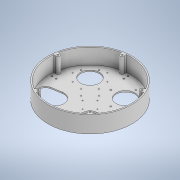
# Autodesk Inventor part: RL_spider_center_mid_v3
Saved by Autodesk Inventor 2022 (Build 260153000, 153)
## iProperties
Created: 2021-08-09
Part Number: RL_spider_center_mid_v3
Material: Generic
Document SubType Name: Modeling
Designer: james
Density: 1 g/cm^3
Appearance: Default
Author: james
Autodesk Inventor part; units mm, degrees
ref_plane "YZ Plane" through (0, 0, 0) normal (1, 0, 0) x (0, 1, 0)
ref_plane "XZ Plane" through (0, 0, 0) normal (0, 1, 0) x (-1, 0, 0)
ref_plane "XY Plane" through (0, 0, 0) normal (0, 0, 1) x (1, 0, 0)
sketch "Sketch1" plane through (0, 0, 0) normal (0, 1, 0) x (-1, 0, 0)
  circle A0 centre (0, 0) radius 100
  dimension "d0" = 200
  constraints: 1 centre point, 1 coincident
  measures "d0" diameter of A0
extrude "Extrusion1" add sketch "Sketch1" along normal blind 40
sketch "Sketch3" plane through (0, 40, 0) normal (0, 1, 0) x (1, 0, 0)
  circle A0 centre (0, 0) radius 97
  circle A1 centre (0, 0) radius 100 projected
  dimension "d14" = 3
  constraints: 1 centre point, 1 coincident
  measures "d14" radial gap between concentric circles of A0 A1
extrude "Extrusion3" cut sketch "Sketch3" against normal blind 37 contours A0
sketch "Sketch6" plane through (0, 40, 0) normal (0, 1, 0) x (1, 0, 0)
  circle A0 centre (65.0538, -65.0538) radius 2.2
  line L0 (0, 0) -> (65.0538, -65.0538)
  line L1 (0, 0) -> (0, 29.3697)
  arc A1 (68.5894, -61.5183) -> (61.5183, -68.5894) centre (65.0538, -65.0538) ccw
  line L2 (61.5183, -68.5894) -> (64.9626, -72.0337)
  line L3 (68.5894, -61.5183) -> (72.0337, -64.9626)
  arc A2 (79.7026, 46.2222) -> (84.2426, 37.3121) centre (81.9726, 41.7671) ccw
  circle A3 centre (81.9726, 41.7671) radius 2.2
  line L4 (84.2426, 37.3121) -> (88.5827, 39.5235)
  line L5 (79.7026, 46.2222) -> (84.0428, 48.4336)
  arc A4 (-19.3304, 90.0852) -> (-9.4535, 91.6495) centre (-14.392, 90.8673) ccw
  circle A5 centre (-14.392, 90.8673) radius 2.2
  line L6 (-9.4535, 91.6495) -> (-10.2155, 96.4606)
  line L7 (-19.3304, 90.0852) -> (-20.0924, 94.8962)
  arc A6 (-91.6495, 9.4535) -> (-90.0852, 19.3304) centre (-90.8673, 14.392) ccw
  circle A7 centre (-90.8673, 14.392) radius 2.2
  line L8 (-90.0852, 19.3304) -> (-94.8962, 20.0924)
  line L9 (-91.6495, 9.4535) -> (-96.4606, 10.2155)
  arc A8 (-37.3121, -84.2426) -> (-46.2222, -79.7026) centre (-41.7671, -81.9726) ccw
  circle A9 centre (-41.7671, -81.9726) radius 2.2
  line L10 (-46.2222, -79.7026) -> (-48.4336, -84.0428)
  line L11 (-37.3121, -84.2426) -> (-39.5235, -88.5827)
  circle A10 centre (0, 0) radius 97 projected
  dimension "d106" = 4.4
  dimension "d109" = 92
  dimension "d111" = 135
  dimension "d112" = 10
  dimension "d115" = 360
  constraints: 24 end point, 10 centre point, 10 point on circle, 2 coincident, 2 parallel, 2 tangent, 1 vertical, 52 other
  measures "d106" diameter of A0
  measures "d109" distance of A0.centre L0.start
  measures "d111" angle of L0 L1
  measures "d112" diameter of A1
extrude "Extrusion6" add sketch "Sketch6" against normal up to surface (37 mm away) contours A1 L3 A10 L2 | A10 L10 A8 L11 | L4 A2 L5 A10 | A10 L8 A6 L9 | L6 A4 L7 A10
sketch "Sketch9" plane through (0, 3, 0) normal (0, 1, 0) x (1, 0, 0)
  circle A0 centre (37.4767, 71.4178) radius 1.75
  circle A1 centre (7.7782, 41.7193) radius 1.75
  circle A2 centre (71.4178, 37.4767) radius 1.75
  circle A3 centre (41.7193, 7.7782) radius 1.75
  line L0 (0, 0) -> (0, 0)
  line L1 (0, 0) -> (-23.1827, 0)
  line L2 (0, 0) -> (0, 0)
  dimension "d115" = 360
  dimension "d77" = 42
  dimension "d78" = 48
  dimension "d79" = 42
  dimension "d80" = 48
  dimension "d81" = 135
  dimension "d82" = 24
  dimension "d83" = 24
  dimension "d84" = 24
  dimension "d85" = 3.5
  dimension "d86" = 3.5
  dimension "d87" = 3.5
  dimension "d88" = 3.5
  dimension "d89" = 35
  constraints: 6 end point, 4 centre point, 1 horizontal, 1 perpendicular
  measures "d77" distance of A1.centre A0.centre
  measures "d78" distance of A3.centre A1.centre
  measures "d79" distance of A3.centre A2.centre
  measures "d80" distance of A2.centre A0.centre
  measures "d81" angle of L0 L1
  measures "d82" distance from line of L0 A1.centre
  measures "d83" distance from line of A3.centre L0
  measures "d84" distance from line of L0 A0.centre
  measures "d85" diameter of A1
  measures "d86" diameter of A3
  measures "d87" diameter of A0
  measures "d88" diameter of A2
  measures "d89" distance from line of L2 A1.centre
extrude "Extrusion9" cut sketch "Sketch9" against normal blind 4
sketch "Sketch18" plane through (0, 3, 0) normal (0, 1, 0) x (1, 0, 0)
  line L0 (54.624, -13.2583) -> (13.2583, -54.624)
  line L1 (13.2583, -54.624) -> (31.643, -73.0088)
  line L2 (31.643, -73.0088) -> (73.0088, -31.643)
  line L3 (73.0088, -31.643) -> (54.624, -13.2583)
  line L4 (0, 0) -> (3.812, 0)
  line L5 (0, 0) -> (33.9411, -33.9411)
  circle A0 centre (54.624, -13.2583) radius 1.15
  circle A1 centre (73.0088, -31.643) radius 1.15
  circle A2 centre (13.2583, -54.624) radius 1.15
  circle A3 centre (31.643, -73.0088) radius 1.15
  line L6 (3.5355, -49.4975) -> (36.7696, -82.7315)
  line L7 (36.7696, -82.7315) -> (82.7315, -36.7696)
  line L8 (82.7315, -36.7696) -> (49.4975, -3.5355)
  line L9 (49.4975, -3.5355) -> (3.5355, -49.4975)
  dimension "d193" = 45
  dimension "d194" = 2.3
  dimension "d195" = 2.3
  dimension "d196" = 2.3
  dimension "d197" = 2.3
  dimension "d198" = 48
  dimension "d199" = 26
  dimension "d200" = 58.5
  dimension "d201" = 47
  dimension "d202" = 10.5
  dimension "d203" = 65
  dimension "d204" = 32.5
  constraints: 20 end point, 7 perpendicular, 4 centre point, 4 coincident, 1 horizontal, 1 midpoint
  measures "d193" angle of L4 L5
  measures "d194" diameter of A0
  measures "d195" diameter of A1
  measures "d196" diameter of A2
  measures "d197" diameter of A3
  measures "d198" distance of L4.start L5.end
  measures "d199" distance of L2.end L0.start
  measures "d200" distance of L1.end L2.end
  measures "d201" distance of L6.start L6.end
  measures "d202" distance between parallel lines of L0 L9
  measures "d203" distance of L8.end L6.start
  measures "d204" distance between parallel lines of L5 L6
extrude "Extrusion11" cut sketch "Sketch18" against normal blind 10 contours L3 A0 L0 | L0 A0 L3 | A1 L2 L3 | L3 L2 A1 | A2 L1 L0 | L0 L1 A2 | A3 L1 L2 | L2 L1 A3
sketch "Sketch12" plane through (0, 3, 0) normal (0, 1, 0) x (1, 0, 0)
  circle A0 centre (-73.0088, 31.643) radius 1.15
  circle A1 centre (-54.624, 13.2583) radius 1.15
  circle A2 centre (-31.643, 73.0088) radius 1.15
  circle A3 centre (-13.2583, 54.624) radius 1.15
  line L0 (-54.624, 13.2583) -> (-73.0088, 31.643)
  line L1 (-73.0088, 31.643) -> (-31.643, 73.0088)
  line L2 (-31.643, 73.0088) -> (-13.2583, 54.624)
  line L3 (-13.2583, 54.624) -> (-54.624, 13.2583)
  line L4 (0, 0) -> (-33.9411, 33.9411)
  line L5 (0, 0) -> (28.9474, 0)
  line L6 (-3.5355, 49.4975) -> (-49.4975, 3.5355)
  line L7 (-49.4975, 3.5355) -> (-82.7315, 36.7696)
  line L8 (-82.7315, 36.7696) -> (-36.7696, 82.7315)
  line L9 (-36.7696, 82.7315) -> (-3.5355, 49.4975)
  dimension "d132" = 135
  dimension "d133" = 58.5
  dimension "d134" = 26
  dimension "d135" = 48
  dimension "d138" = 2.3
  dimension "d139" = 2.3
  dimension "d140" = 2.3
  dimension "d141" = 2.3
  dimension "d219" = 47
  dimension "d220" = 65
  dimension "d221" = 32.5
  dimension "d222" = 10.5
  constraints: 20 end point, 7 perpendicular, 4 centre point, 1 horizontal, 1 midpoint, 1 parallel
  measures "d132" angle of L4 L5
  measures "d133" distance of L2.end L0.start
  measures "d134" distance of L0.start L0.end
  measures "d135" distance of L4.start L4.end
  measures "d138" diameter of A1
  measures "d139" diameter of A0
  measures "d140" diameter of A3
  measures "d141" diameter of A2
  measures "d219" distance of L6.end L7.end
  measures "d220" distance of L6.start L6.end
  measures "d221" distance between parallel lines of L4 L7
  measures "d222" distance between parallel lines of L6 L3
extrude "Extrusion12" cut sketch "Sketch12" against normal blind 10 contours A0 L0 L1 | L1 L0 A0 | L1 L2 A2 | A2 L2 L1 | L0 L3 A1 | A1 L3 L0 | L2 L3 A3 | A3 L3 L2
sketch "Sketch13" plane through (0, 3, 0) normal (0, 1, 0) x (1, 0, 0)
  circle A0 centre (-3.8891, -13.7886) radius 1.15
  circle A1 centre (13.7886, 3.8891) radius 1.15
  circle A2 centre (13.7886, -31.4663) radius 1.15
  circle A3 centre (31.4663, -13.7886) radius 1.15
  line L0 (13.7886, 3.8891) -> (31.4663, -13.7886)
  line L1 (13.7886, 3.8891) -> (-3.8891, -13.7886)
  line L2 (-3.8891, -13.7886) -> (13.7886, -31.4663)
  line L3 (13.7886, -31.4663) -> (31.4663, -13.7886)
  line L4 (0, 0) -> (4.9497, -4.9497)
  line L5 (0, 0) -> (0, 15.8788)
  circle A4 centre (-54.624, 13.2583) radius 1.15 projected
  circle A5 centre (-13.2583, 54.624) radius 1.15 projected
  line L6 (-54.624, 13.2583) -> (-13.2583, 54.624)
  dimension "d142" = 25
  dimension "d143" = 25
  dimension "d146" = 7
  dimension "d147" = 2.3
  dimension "d148" = 2.3
  dimension "d149" = 2.3
  dimension "d150" = 2.3
  dimension "d218" = 225
  constraints: 14 end point, 4 centre point, 4 perpendicular, 1 midpoint, 1 vertical
  measures "d142" distance of L0.start L1.end
  measures "d143" distance of L0.start L0.end
  measures "d146" distance of L4.start L4.end
  measures "d147" diameter of A1
  measures "d148" diameter of A3
  measures "d149" diameter of A2
  measures "d150" diameter of A0
extrude "Extrusion13" cut sketch "Sketch13" against normal blind 10 contours A0 L2 L1 | L1 L2 A0 | L2 L3 A2 | A2 L3 L2 | L1 L0 A1 | A1 L0 L1 | L3 L0 A3 | A3 L0 L3
sketch "Sketch14" plane through (0, 3, 0) normal (0, 1, 0) x (1, 0, 0)
  circle A0 centre (-15.5563, -5.6569) radius 1.15
  circle A1 centre (-29.6985, 8.4853) radius 1.15
  circle A2 centre (5.6569, 15.5563) radius 1.15
  circle A3 centre (-8.4853, 29.6985) radius 1.15
  line L0 (-15.5563, -5.6569) -> (-29.6985, 8.4853)
  line L1 (-29.6985, 8.4853) -> (-8.4853, 29.6985)
  line L2 (-8.4853, 29.6985) -> (5.6569, 15.5563)
  line L3 (5.6569, 15.5563) -> (-15.5563, -5.6569)
  line L4 (0, 0) -> (-4.9497, 4.9497)
  line L5 (0, 0) -> (0, -29.7701)
  circle A4 centre (13.2583, -54.624) radius 1.15 projected
  circle A5 centre (54.624, -13.2583) radius 1.15 projected
  line L6 (13.2583, -54.624) -> (54.624, -13.2583)
  dimension "d153" = 20
  dimension "d154" = 30
  dimension "d155" = 2.3
  dimension "d156" = 2.3
  dimension "d157" = 2.3
  dimension "d158" = 2.3
  dimension "d160" = 7
  dimension "d217" = 225
  constraints: 14 end point, 4 centre point, 4 perpendicular, 1 midpoint, 1 vertical
  measures "d153" distance of L0.start L0.end
  measures "d154" distance of L2.end L0.start
  measures "d155" diameter of A2
  measures "d156" diameter of A3
  measures "d157" diameter of A0
  measures "d158" diameter of A1
  measures "d160" distance of L4.start L4.end
extrude "Extrusion14" cut sketch "Sketch14" against normal blind 10 contours A0 L0 L3 | L3 L0 A0 | L0 L1 A1 | A1 L1 L0 | L3 L2 A2 | A2 L2 L3 | L1 L2 A3 | A3 L2 L1
sketch "Sketch16" plane through (0, 3, 0) normal (0, 1, 0) x (1, 0, 0)
  circle A0 centre (0, 80.5) radius 1.75
  circle A1 centre (0, 90.5) radius 1.75
  circle A2 centre (0, 0) radius 100 projected
  line L0 (0, 100) -> (0, 80.5)
  dimension "d179" = 3.5
  dimension "d180" = 19.5
  dimension "d181" = 9.5
  dimension "d182" = 3.5
  constraints: 2 centre point, 2 end point, 1 vertical, 1 vertical alignment, 1 other
  measures "d179" diameter of A0
  measures "d180" distance of L0.start L0.end
  measures "d181" distance of A1.centre L0.start
  measures "d182" diameter of A1
extrude "Extrusion16" cut sketch "Sketch16" against normal blind 10 contours A0 | A1 L0 | L0 A1
pattern_circular "Circular Pattern4" count 4 over 360 about axis through (0, -10, 0) along (0, 1, 0) of "Extrusion16"
sketch "Sketch17" plane through (0, 3, 0) normal (0, 1, 0) x (1, 0, 0)
  line L0 (0, 0) -> (-53.033, -53.033)
  line L1 (-53.033, -53.033) -> (-67.1751, -38.8909)
  line L2 (0, 0) -> (-22.9121, 0)
  line L3 (0, 0) -> (-42.4264, 42.4264)
  circle A0 centre (-42.4264, 42.4264) radius 22.5
  circle A1 centre (-42.4264, -42.4264) radius 22.5
  circle A2 centre (42.4264, -42.4264) radius 22.5
  circle A3 centre (42.4264, 42.4264) radius 22.5
  line L4 (-69.6063, -24.0892) -> (-46.0732, -20.2239)
  line L5 (-73.6535, -52.4198) -> (-52.144, -62.7197)
  arc A4 (-69.6063, -24.0892) -> (-73.6535, -52.4198) centre (-67.1751, -38.8909) ccw
  point P0 (-64.8915, -41.1745)
  point P1 (-26.5165, -26.5165)
  dimension "d188" = 45
  dimension "d189" = 75
  dimension "d190" = 20
  dimension "d207" = 60
  dimension "d208" = 45
  dimension "d209" = 45
  dimension "d212" = 360
  dimension "d216" = 15
  constraints: 12 end point, 5 centre point, 4 point on circle, 4 tangent, 2 coincident, 1 horizontal, 1 perpendicular, 9 other
  measures "d188" angle of L0 L2
  measures "d189" distance of L0.start L0.end
  measures "d190" distance of L0.end L1.end
  measures "d207" distance of L0.start L3.end
  measures "d208" diameter of A0
  measures "d209" angle of L2 L3
  measures "d216" radius of A4
extrude "Extrusion18" cut sketch "Sketch17" against normal blind 10
sketch "Sketch20" plane through (0, 3, 0) normal (0, 1, 0) x (1, 0, 0)
  line L0 (0, 0) -> (-22.6274, 22.6274)
  line L1 (-22.6274, 22.6274) -> (-29.7758, 15.479)
  line L2 (-22.6274, 22.6274) -> (-15.6337, 29.6211)
  line L3 (0, 0) -> (9.6667, 0)
  circle A0 centre (-29.7758, 15.479) radius 1.75
  circle A1 centre (-15.6337, 29.6211) radius 1.75
  circle A2 centre (-68.5894, 47.3762) radius 1.75
  circle A3 centre (-47.3762, 68.5894) radius 1.75
  line L4 (-68.5894, 47.3762) -> (-47.3762, 68.5894)
  line L5 (-57.9828, 57.9828) -> (-22.6274, 22.6274)
  dimension "d223" = 135
  dimension "d224" = 3.5
  dimension "d225" = 3.5
  dimension "d226" = 20
  dimension "d227" = 32
  dimension "d228" = 30
  dimension "d229" = 3.5
  dimension "d230" = 3.5
  dimension "d231" = 50
  constraints: 12 end point, 4 centre point, 3 perpendicular, 2 coincident, 1 collinear, 1 horizontal, 1 midpoint
  measures "d223" angle of L3 L0
  measures "d224" diameter of A0
  measures "d225" diameter of A1
  measures "d226" distance of L2.end L1.end
  measures "d227" distance of L0.start L0.end
  measures "d228" distance of L4.start L4.end
  measures "d229" diameter of A3
  measures "d230" diameter of A2
  measures "d231" distance of L5.start L0.end
extrude "Extrusion19" cut sketch "Sketch20" against normal blind 10 contours A2 | A3
body "Solid1"
